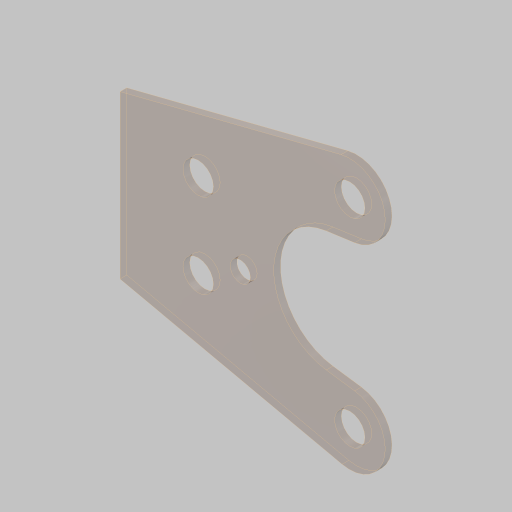
# Autodesk Inventor part: Part1
Saved by Autodesk Inventor 2023.5 (Build 275446000, 446)
## iProperties
Created: 2025-02-23
Part Number: Part1
Material: Polycarbonate, Smoke
Document SubType Name: Modeling
Designer: slick
Density: 1.2 g/cm^3
Appearance: Polycarbonate - Smoked
Author: slick
Autodesk Inventor part; units mm, degrees
ref_plane "YZ Plane" through (0, 0, 0) normal (1, 0, 0) x (0, 1, 0)
ref_plane "XZ Plane" through (0, 0, 0) normal (0, 1, 0) x (-1, 0, 0)
ref_plane "XY Plane" through (0, 0, 0) normal (0, 0, 1) x (1, 0, 0)
sketch "Sketch1" plane through (0, 0, 0) normal (0, 0, 1) x (1, 0, 0)
  circle A0 centre (0, 93.3256) radius 38.1 construction
  circle A1 centre (0, -93.3256) radius 38.1 construction
  line L0 (0, 93.3256) -> (0, -93.3256) construction
  circle A2 centre (-19.05, 0) radius 57.15 construction
  circle A3 centre (0, 93.3256) radius 14.2875
  circle A4 centre (0, -93.3256) radius 14.2875
  circle A5 centre (0, -93.3256) radius 33.3375 construction
  circle A6 centre (0, 93.3256) radius 33.3375 construction
  circle A7 centre (-142.4318, -39.6875) radius 14.3256 construction
  circle A8 centre (0, -93.3256) radius 23.876 construction
  line L1 (-142.4318, -39.6875) -> (0, -93.3256) construction
  circle A9 centre (-142.4318, 39.6875) radius 14.3256 construction
  circle A10 centre (0, 93.3256) radius 23.876 construction
  line L2 (0, 93.3256) -> (-142.4318, 39.6875) construction
  circle A11 centre (-142.4318, 39.6875) radius 39.6875 construction
  circle A12 centre (-142.4318, -39.6875) radius 39.6875 construction
  line L3 (-142.4318, 39.6875) -> (-142.4318, -39.6875) construction
  line L4 (-138.2343, 25.9906) -> (6.9958, 70.4975) construction
  line L5 (-9.8, 115.0976) -> (-148.3118, 52.7507) construction
  line L6 (-138.2343, -25.9906) -> (6.9958, -70.4975) construction
  line L7 (-9.8, -115.0976) -> (-148.3118, -52.7507) construction
  circle A13 centre (-142.4318, 39.6875) radius 14.2875
  circle A14 centre (-142.4318, -39.6875) radius 14.2875
  circle A15 centre (-102.9059, -16.8672) radius 5.9531 construction
  circle A16 centre (-102.9059, -16.8672) radius 9.525
  circle A17 centre (-102.9059, -16.8672) radius 12.7 construction
  circle A18 centre (-102.9059, -16.8672) radius 12.7 construction
  circle A19 centre (-102.9059, -16.8672) radius 12.7 construction
  circle A20 centre (-102.9059, -16.8672) radius 12.7 construction
  circle A21 centre (-102.9059, -16.8672) radius 12.7 construction
  circle A22 centre (-14.2875, 0) radius 57.15 construction
  circle A23 centre (-102.9059, -16.8672) radius 19.05 construction
  line L8 (-215.9, 73.025) -> (-190.5, 73.025) construction
  line L9 (-190.5, 73.025) -> (-190.5, -79.375) construction
  line L10 (-190.5, -79.375) -> (-215.9, -79.375) construction
  line L11 (-215.9, -79.375) -> (-215.9, 73.025)
  line L12 (-142.4318, -39.6875) -> (-102.9059, -16.8672) construction
  line L13 (-79.1995, 63.5) -> (-79.1995, -63.5) construction
  line L14 (-215.9, 73.025) -> (-8.1864, 125.6423)
  line L15 (-215.9, -79.375) -> (-7.2503, -125.8651)
  line L16 (-22.1185, -56.6109) -> (4.5681, -60.3025)
  arc A24 (4.5681, 60.3025) -> (-8.1864, 125.6423) centre (0, 93.3256) ccw
  arc A25 (-22.1185, 56.6109) -> (-22.1185, -56.6109) centre (-14.2875, 0) ccw
  line L17 (4.5681, 60.3025) -> (-22.1185, 56.6109)
  arc A26 (-7.2503, -125.8651) -> (4.5681, -60.3025) centre (0, -93.3256) ccw
  point P0 (0, 0)
  point P1 (0, 0)
  point P2 (-111.0402, -7.1141)
  point P3 (-114.6953, -21.5895)
  point P4 (-102.0579, -29.5388)
  point P5 (-90.5924, -19.9764)
  point P6 (-96.1437, -6.1171)
  dimension "d15" = 25.4
  dimension "d0" = 76.2
  dimension "d1" = 76.2
  dimension "d2" = 114.3
  dimension "d3" = 19.05
  dimension "d4" = 186.6511
  dimension "d5" = 28.575
  dimension "d6" = 19.05
  dimension "d7" = 28.6512
  dimension "d8" = 47.752
  dimension "d9" = 79.375
  dimension "d10" = 142.4318
  dimension "d11" = 152.1968
  dimension "d12" = 28.575
  dimension "d13" = 11.9062
  dimension "d14" = 19.05
  dimension "d18" = 360
  dimension "d20" = 4.7625
  dimension "d21" = 38.1
  dimension "d22" = 25.4
  dimension "d23" = 152.4
  dimension "d24" = 215.9
  dimension "d25" = 60
  dimension "d26" = 127
  constraints: 36 end point, 22 centre point, 20 point on circle, 18 tangent, 15 coincident, 7 equal radius, 3 vertical, 2 parallel, 2 point on line, 1 equal length, 1 horizontal, 1 horizontal alignment, 1 midpoint, 1 perpendicular, 31 other
  measures "d0" diameter of A0
  measures "d1" diameter of A1
  measures "d2" diameter of A2
  measures "d3" distance of point (0, 0) A2.centre
  measures "d4" distance of L0.end L0.start
  measures "d5" diameter of A3
  measures "d6" radial gap between concentric circles of A4 A5
  measures "d7" diameter of A7
  measures "d8" diameter of A8
  measures "d9" diameter of A11
  measures "d10" distance from line of L3 L0.start
  measures "d11" distance of L2.start L2.end
  measures "d12" diameter of A13
  measures "d13" diameter of A15
  measures "d14" diameter of A16
  measures "d20" distance of A2.centre A22.centre
  measures "d21" diameter of A23
  measures "d22" distance of L9.end L10.end
  measures "d23" distance of L10.end L8.start
  measures "d24" distance from line of A3.centre L11
  measures "d25" angle of L12 L3
  measures "d26" distance of L13.start L13.end
extrude "Extrusion1" add sketch "Sketch1" along normal mid plane 6.35
body "Solid1"
